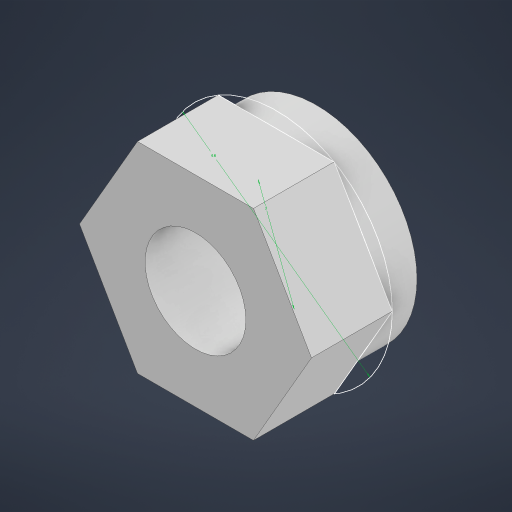
# Autodesk Inventor part: m2_locknut
Saved by Autodesk Inventor 2023 (Build 270158000, 158)
## iProperties
Created: 2024-02-24
Part Number: m2_locknut
Material: 一般
Document SubType Name: Modeling
Designer: MasakatsuHonda
Density: 1 g/cm^3
Appearance: 既定
Author: MasakatsuHonda
Autodesk Inventor part; units mm, degrees
ref_plane "YZ Plane" through (0, 0, 0) normal (1, 0, 0) x (0, 1, 0)
ref_plane "XZ Plane" through (0, 0, 0) normal (0, 1, 0) x (-1, 0, 0)
ref_plane "XY Plane" through (0, 0, 0) normal (0, 0, 1) x (1, 0, 0)
sketch "スケッチ1" plane through (0, 0, 0) normal (0, 0, 1) x (1, 0, 0)
  circle A0 centre (0, 0) radius 2.3
  line L0 (1.15, 1.9919) -> (2.3, 0)
  line L1 (2.3, 0) -> (1.15, -1.9919)
  line L2 (1.15, -1.9919) -> (-1.15, -1.9919)
  line L3 (-1.15, -1.9919) -> (-2.3, 0)
  line L4 (-2.3, 0) -> (-1.15, 1.9919)
  line L5 (-1.15, 1.9919) -> (1.15, 1.9919)
  circle A1 centre (0, 0) radius 1
  circle A2 centre (0, 0) radius 1.9919
  dimension "d0" = 4.6
  dimension "d1" = 2
  constraints: 12 end point, 4 coincident, 2 centre point, 1 horizontal, 1 tangent, 16 other
  measures "d1" diameter of A1
extrude "押し出し1" add sketch "スケッチ1" along normal blind 1.6 contours L1 A2 L0 | L0 A2 L5 | L2 A2 L1 | A2 | L5 A2 L4 | L3 A2 L2 | L4 A2 L3
extrude "押し出し2" add sketch "スケッチ1" against normal blind 0.8 contours A2
